X306_Panel (Autodesk Fusion 360 design; units mm, degrees)
part number: 2026-07-25-11-08-38-963
Autodesk Fusion 360 part; units mm, degrees
note: some values were not read from the file. Chosen so that the rebuilt part matches the saved one: which bodies a step acts on.
sketch "Sketch197" plane through (0, 0, 0) normal (0, 0, 1) x (1, 0, 0)
  line L0 (-43.7, -31.15) -> (43.7, -31.15)
  line L1 (43.7, -31.15) -> (43.7, 31.15)
  line L2 (43.7, 31.15) -> (-43.7, 31.15)
  line L3 (-43.7, 31.15) -> (-43.7, -31.15)
extrude "Extrude197" add sketch "Sketch197" along normal blind 5 makes body 1
ref_plane "WorkPlane11" through (0, 0, 5) normal (0, 0, 1) x (1, 0, 0)
sketch "Sketch198" plane through (0, 0, 5) normal (0, 0, 1) x (1, 0, 0)
  line L0 (-38.7, -26.15) -> (38.7, -26.15)
  line L1 (38.7, -26.15) -> (38.7, 26.15)
  line L2 (38.7, 26.15) -> (-38.7, 26.15)
  line L3 (-38.7, 26.15) -> (-38.7, -26.15)
extrude "Extrude198" cut sketch "Sketch198" against normal blind 2 bodies 1
sketch "Sketch199" plane through (0, 0, 0) normal (0, 0, 1) x (1, 0, 0)
  circle A0 centre (-35.05, 0.5) radius 1.55
extrude "Extrude199" cut sketch "Sketch199" along normal blind 6 bodies 1
sketch "Sketch200" plane through (0, 0, 0) normal (0, 0, 1) x (1, 0, 0)
  circle A0 centre (-35.05, -22.5) radius 1.55
extrude "Extrude200" cut sketch "Sketch200" along normal blind 6 bodies 1
sketch "Sketch201" plane through (0, 0, 0) normal (0, 0, 1) x (1, 0, 0)
  circle A0 centre (22.95, 0.5) radius 1.55
extrude "Extrude201" cut sketch "Sketch201" along normal blind 6 bodies 1
sketch "Sketch202" plane through (0, 0, 0) normal (0, 0, 1) x (1, 0, 0)
  circle A0 centre (22.95, -22.5) radius 1.55
extrude "Extrude202" cut sketch "Sketch202" along normal blind 6 bodies 1
ref_plane "WorkPlane12" through (0, 0, 5) normal (0, 0, 1) x (1, 0, 0)
sketch "Sketch203" plane through (0, 0, 5) normal (0, 0, 1) x (1, 0, 0)
  line L0 (-44.7, -16.03) -> (-38.7, -16.03)
  line L1 (-38.7, -16.03) -> (-38.7, -8.03)
  line L2 (-38.7, -8.03) -> (-44.7, -8.03)
  line L3 (-44.7, -8.03) -> (-44.7, -16.03)
extrude "Extrude203" cut sketch "Sketch203" against normal blind 2 bodies 1
ref_plane "WorkPlane13" through (0, 0, 1.4) normal (0, 0, 1) x (1, 0, 0)
sketch "Sketch204" plane through (0, 0, 0) normal (0, 0, 1) x (1, 0, 0)
  circle A0 centre (-35.05, 0.5) radius 2.95
sketch "Sketch205" plane through (0, 0, 1.4) normal (0, 0, 1) x (1, 0, 0)
  circle A0 centre (-35.05, 0.5) radius 1.55
loft "Loft1" cut profiles "Sketch204", "Sketch205" section 1 section 2 bodies 1
sketch "Sketch206" plane through (0, 0, 0) normal (0, 0, 1) x (1, 0, 0)
  circle A0 centre (-35.05, -22.5) radius 2.95
sketch "Sketch207" plane through (0, 0, 1.4) normal (0, 0, 1) x (1, 0, 0)
  circle A0 centre (-35.05, -22.5) radius 1.55
loft "Loft2" cut profiles "Sketch206", "Sketch207" section 1 section 2 bodies 1
sketch "Sketch208" plane through (0, 0, 0) normal (0, 0, 1) x (1, 0, 0)
  circle A0 centre (22.95, 0.5) radius 2.95
sketch "Sketch209" plane through (0, 0, 1.4) normal (0, 0, 1) x (1, 0, 0)
  circle A0 centre (22.95, 0.5) radius 1.55
loft "Loft3" cut profiles "Sketch208", "Sketch209" section 1 section 2 bodies 1
sketch "Sketch210" plane through (0, 0, 0) normal (0, 0, 1) x (1, 0, 0)
  circle A0 centre (22.95, -22.5) radius 2.95
sketch "Sketch211" plane through (0, 0, 1.4) normal (0, 0, 1) x (1, 0, 0)
  circle A0 centre (22.95, -22.5) radius 1.55
loft "Loft4" cut profiles "Sketch210", "Sketch211" section 1 section 2 bodies 1
ref_plane "WorkPlane14" through (0, 0, 5) normal (0, 0, 1) x (1, 0, 0)
sketch "Sketch212" plane through (0, 0, 5) normal (0, 0, 1) x (1, 0, 0)
  line L0 (27.25, -32.15) -> (37.25, -32.15)
  line L1 (37.25, -32.15) -> (37.25, -26.15)
  line L2 (37.25, -26.15) -> (27.25, -26.15)
  line L3 (27.25, -26.15) -> (27.25, -32.15)
extrude "Extrude204" cut sketch "Sketch212" against normal blind 2 bodies 1
ref_plane "WorkPlane15" through (0, 0, 3) normal (0, 0, 1) x (1, 0, 0)
sketch "Sketch213" plane through (0, 0, 3) normal (0, 0, 1) x (1, 0, 0)
  circle A0 centre (-36.405, 15.35) radius 1
extrude "Extrude205" cut sketch "Sketch213" against normal blind 2 bodies 1
sketch "Sketch214" plane through (0, 0, 3) normal (0, 0, 1) x (1, 0, 0)
  circle A0 centre (36.405, 15.35) radius 1
extrude "Extrude206" cut sketch "Sketch214" against normal blind 2 bodies 1
ref_plane "WorkPlane16" through (0, 0, 3) normal (0, 0, 1) x (1, 0, 0)
sketch "Sketch215" plane through (0, 0, 3) normal (0, 0, 1) x (1, 0, 0)
  circle A0 centre (-27.6, 7.35) radius 1.825
extrude "Extrude207" cut sketch "Sketch215" against normal blind 2 bodies 1
sketch "Sketch216" plane through (0, 0, 3) normal (0, 0, 1) x (1, 0, 0)
  circle A0 centre (27.6, 23.35) radius 1.825
extrude "Extrude208" cut sketch "Sketch216" against normal blind 2 bodies 1
ref_plane "WorkPlane17" through (0, 0, 5) normal (0, 0, 1) x (1, 0, 0)
sketch "Sketch217" plane through (0, 0, 5) normal (0, 0, 1) x (1, 0, 0)
  line L0 (-43.7, -31.15) -> (43.7, -31.15)
  line L1 (43.7, -31.15) -> (43.7, 31.15)
  line L2 (43.7, 31.15) -> (-43.7, 31.15)
  line L3 (-43.7, 31.15) -> (-43.7, -31.15)
extrude "Extrude209" add sketch "Sketch217" along normal blind 20 separate body makes body 2
sketch "Sketch218" plane through (0, 0, 5) normal (0, 0, 1) x (1, 0, 0)
  line L0 (-38.7, -26.15) -> (38.7, -26.15)
  line L1 (38.7, -26.15) -> (38.7, 26.15)
  line L2 (38.7, 26.15) -> (-38.7, 26.15)
  line L3 (-38.7, 26.15) -> (-38.7, -26.15)
extrude "Extrude210" cut sketch "Sketch218" along normal blind 20 bodies 2
sketch "Sketch219" plane through (0, 0, 5) normal (0, 0, 1) x (1, 0, 0)
  line L0 (-44.7, -16.03) -> (-37.7, -16.03)
  line L1 (-37.7, -16.03) -> (-37.7, -8.03)
  line L2 (-37.7, -8.03) -> (-44.7, -8.03)
  line L3 (-44.7, -8.03) -> (-44.7, -16.03)
extrude "Extrude211" cut sketch "Sketch219" along normal blind 20 bodies 2
sketch "Sketch220" plane through (0, 0, 5) normal (0, 0, 1) x (1, 0, 0)
  line L0 (27.25, -32.65) -> (37.25, -32.65)
  line L1 (37.25, -32.65) -> (37.25, -25.65)
  line L2 (37.25, -25.65) -> (27.25, -25.65)
  line L3 (27.25, -25.65) -> (27.25, -32.65)
extrude "Extrude212" cut sketch "Sketch220" along normal blind 20 bodies 2 makes body 3 at (-20.05, -31.15, 18.3333)
combine "Combine8" operation add target body 1 tool bodies 2
combine "Combine9" operation add target body 1 tool bodies 3
ref_plane "WorkPlane18" through (0, 0, 3) normal (0, 0, 1) x (1, 0, 0)
sketch "Sketch221" plane through (0, 0, 3) normal (0, 0, 1) x (1, 0, 0)
  line L0 (25.25, -32.15) -> (39.25, -32.15)
  line L1 (39.25, -32.15) -> (39.25, -26.15)
  line L2 (39.25, -26.15) -> (25.25, -26.15)
  line L3 (25.25, -26.15) -> (25.25, -32.15)
extrude "Extrude213" cut sketch "Sketch221" along normal blind 22 bodies 1
ref_plane "WorkPlane19" through (0, 0, 9) normal (0, 0, 1) x (1, 0, 0)
sketch "Sketch222" plane through (0, 0, 9) normal (0, 0, 1) x (1, 0, 0)
  line L0 (-43.7, -16.03) -> (-38.7, -16.03)
  line L1 (-38.7, -16.03) -> (-38.7, -8.03)
  line L2 (-38.7, -8.03) -> (-43.7, -8.03)
  line L3 (-43.7, -8.03) -> (-43.7, -16.03)
extrude "Extrude214" add sketch "Sketch222" along normal blind 16 separate body makes body 4
ref_plane "WorkPlane20" through (0, 0, 11) normal (0, 0, 1) x (1, 0, 0)
sketch "Sketch223" plane through (0, 0, 11) normal (0, 0, 1) x (1, 0, 0)
  line L0 (25.25, -31.15) -> (39.25, -31.15)
  line L1 (39.25, -31.15) -> (39.25, -26.15)
  line L2 (39.25, -26.15) -> (25.25, -26.15)
  line L3 (25.25, -26.15) -> (25.25, -31.15)
extrude "Extrude215" add sketch "Sketch223" along normal blind 14 separate body makes body 5
combine "Combine10" operation add target body 1 tool bodies 4 5
ref_plane "WorkPlane21" through (0, 0, 3) normal (0, 0, 1) x (1, 0, 0)
sketch "Sketch224" plane through (0, 0, 3) normal (0, 0, 1) x (1, 0, 0)
  line L0 (-38.7, -26.15) -> (-35.5, -26.15)
  line L1 (-35.5, -26.15) -> (-38.7, -22.95)
  line L2 (-38.7, -22.95) -> (-38.7, -26.15)
extrude "Extrude216" cut sketch "Sketch224" along normal blind 22 bodies 1
sketch "Sketch225" plane through (0, 0, 3) normal (0, 0, 1) x (1, 0, 0)
  line L0 (38.7, -26.15) -> (35.5, -26.15)
  line L1 (35.5, -26.15) -> (38.7, -22.95)
  line L2 (38.7, -22.95) -> (38.7, -26.15)
extrude "Extrude217" cut sketch "Sketch225" along normal blind 22 bodies 1
sketch "Sketch226" plane through (0, 0, 3) normal (0, 0, 1) x (1, 0, 0)
  line L0 (-38.7, 26.15) -> (-38, 26.15)
  line L1 (-38, 26.15) -> (-38.7, 25.45)
  line L2 (-38.7, 25.45) -> (-38.7, 26.15)
extrude "Extrude218" cut sketch "Sketch226" along normal blind 22 bodies 1
sketch "Sketch227" plane through (0, 0, 3) normal (0, 0, 1) x (1, 0, 0)
  line L0 (38.7, 26.15) -> (38, 26.15)
  line L1 (38, 26.15) -> (38.7, 25.45)
  line L2 (38.7, 25.45) -> (38.7, 26.15)
extrude "Extrude219" cut sketch "Sketch227" along normal blind 22 bodies 1
ref_plane "WorkPlane22" through (0, 0, 5) normal (0, 0, 1) x (1, 0, 0)
sketch "Sketch228" plane through (0, 0, 5) normal (0, 0, 1) x (1, 0, 0)
  line L0 (-44.7, -31.15) -> (44.7, -31.15)
  line L1 (44.7, -31.15) -> (44.7, -26.15)
  line L2 (44.7, -26.15) -> (-44.7, -26.15)
  line L3 (-44.7, -26.15) -> (-44.7, -31.15)
extrude "Extrude220" cut sketch "Sketch228" along normal blind 20 bodies 1
ref_plane "WorkPlane23" through (0, 0, 5) normal (0, 0, 1) x (1, 0, 0)
sketch "Sketch229" plane through (0, 0, 5) normal (0, 0, 1) x (1, 0, 0)
  line L0 (-43.7, -31.15) -> (-38.7, -31.15)
  line L1 (-38.7, -31.15) -> (-38.7, -26.15)
  line L2 (-38.7, -26.15) -> (-43.7, -26.15)
  line L3 (-43.7, -26.15) -> (-43.7, -31.15)
extrude "Extrude221" add sketch "Sketch229" along normal blind 20 separate body makes body 6
sketch "Sketch230" plane through (0, 0, 5) normal (0, 0, 1) x (1, 0, 0)
  line L0 (38.7, -31.15) -> (43.7, -31.15)
  line L1 (43.7, -31.15) -> (43.7, -26.15)
  line L2 (43.7, -26.15) -> (38.7, -26.15)
  line L3 (38.7, -26.15) -> (38.7, -31.15)
extrude "Extrude222" add sketch "Sketch230" along normal blind 20 separate body makes body 7
combine "Combine11" operation add target body 1 tool bodies 6 7
ref_plane "WorkPlane24" through (0, 0, 3) normal (0, 0, 1) x (1, 0, 0)
sketch "Sketch231" plane through (0, 0, 3) normal (0, 0, 1) x (1, 0, 0)
  line L0 (-43.7, -16.03) -> (-38.7, -16.03)
  line L1 (-38.7, -16.03) -> (-38.7, -8.03)
  line L2 (-38.7, -8.03) -> (-43.7, -8.03)
  line L3 (-43.7, -8.03) -> (-43.7, -16.03)
extrude "Extrude223" add sketch "Sketch231" along normal blind 6 separate body makes body 8
combine "Combine12" operation add target body 1 tool bodies 8
ref_plane "WorkPlane25" through (-43.7, 0, 0) normal (1, 0, 0) x (0, 1, 0)
sketch "Sketch232" plane through (-43.7, 0, 0) normal (1, 0, 0) x (0, 0, -1)
  circle A0 centre (-6, -16.5) radius 3.2
extrude "Extrude224" cut sketch "Sketch232" along normal blind 5.2 bodies 1
sketch "Sketch233" plane through (0, 0, 0) normal (0, 0, 1) x (1, 0, 0)
  line L0 (-49.7, -37.15) -> (-43.7, -37.15)
  line L1 (-43.7, -37.15) -> (-43.7, 37.15)
  line L2 (-43.7, 37.15) -> (-49.7, 37.15)
  line L3 (-49.7, 37.15) -> (-49.7, -37.15)
extrude "Extrude225" add sketch "Sketch233" along normal blind 25 separate body makes body 9
sketch "Sketch234" plane through (0, 0, 0) normal (0, 0, 1) x (1, 0, 0)
  line L0 (43.7, -37.15) -> (49.7, -37.15)
  line L1 (49.7, -37.15) -> (49.7, 37.15)
  line L2 (49.7, 37.15) -> (43.7, 37.15)
  line L3 (43.7, 37.15) -> (43.7, -37.15)
extrude "Extrude226" add sketch "Sketch234" along normal blind 25 separate body makes body 10
sketch "Sketch235" plane through (0, 0, 0) normal (0, 0, 1) x (1, 0, 0)
  line L0 (-43.7, 31.15) -> (43.7, 31.15)
  line L1 (43.7, 31.15) -> (43.7, 37.15)
  line L2 (43.7, 37.15) -> (-43.7, 37.15)
  line L3 (-43.7, 37.15) -> (-43.7, 31.15)
extrude "Extrude227" add sketch "Sketch235" along normal blind 25 separate body makes body 11
sketch "Sketch236" plane through (0, 0, 0) normal (0, 0, 1) x (1, 0, 0)
  line L0 (-43.7, -37.15) -> (43.7, -37.15)
  line L1 (43.7, -37.15) -> (43.7, -31.15)
  line L2 (43.7, -31.15) -> (-43.7, -31.15)
  line L3 (-43.7, -31.15) -> (-43.7, -37.15)
extrude "Extrude228" add sketch "Sketch236" along normal blind 5 separate body makes body 12
combine "Combine13" operation add target body 1 tool bodies 9 10 11 12
ref_plane "WorkPlane27" through (-49.7, 0, 0) normal (1, 0, 0) x (0, 1, 0)
sketch "Sketch238" plane through (-49.7, 0, 0) normal (1, 0, 0) x (0, 0, -1)
  circle A0 centre (-6, -16.5) radius 3.2
extrude "Extrude229" cut sketch "Sketch238" along normal blind 11.3 bodies 1
ref_plane "WorkPlane28" through (0, -37.15, 0) normal (0, 1, 0) x (0, 0, 1)
sketch "Sketch239" plane through (0, -37.15, 0) normal (0, 1, 0) x (1, 0, 0)
  line L0 (25.25, -5) -> (39.25, -5)
  line L1 (39.25, -5) -> (39.25, -3)
  line L2 (39.25, -3) -> (25.25, -3)
  line L3 (25.25, -3) -> (25.25, -5)
extrude "Extrude230" cut sketch "Sketch239" along normal blind 11.2 bodies 1
sketch "Sketch240" plane through (0, 0, 0) normal (0, 0, 1) x (1, 0, 0)
  line L0 (38.7, -37.15) -> (49.7, -37.15)
  line L1 (49.7, -37.15) -> (49.7, -26.15)
  line L2 (49.7, -26.15) -> (38.7, -26.15)
  line L3 (38.7, -26.15) -> (38.7, -37.15)
  line L4 (-49.7, -37.15) -> (-38.7, -37.15)
  line L5 (-38.7, -37.15) -> (-38.7, -26.15)
  line L6 (-38.7, -26.15) -> (-49.7, -26.15)
  line L7 (-49.7, -26.15) -> (-49.7, -37.15)
extrude "Extrude231" add sketch "Sketch240" along normal blind 25 separate body makes body 13 at (46.0333, -26.15, 8.3333) makes body 14 at (-42.3667, -26.15, 8.3333)
combine "Combine14" operation add target body 1 tool bodies 13 14
ref_plane "WorkPlane29" through (0, -37.15, 0) normal (0, 1, 0) x (0, 0, 1)
sketch "Sketch241" plane through (0, -37.15, 0) normal (0, 1, 0) x (1, 0, 0)
  line L0 (25.25, -5) -> (39.25, -5)
  line L1 (39.25, -5) -> (39.25, -3)
  line L2 (39.25, -3) -> (25.25, -3)
  line L3 (25.25, -3) -> (25.25, -5)
extrude "Extrude232" cut sketch "Sketch241" along normal blind 11.2 bodies 1
sketch "Sketch242" plane through (0, 0, 0) normal (0, 0, 1) x (1, 0, 0)
  circle A0 centre (-44.2, 31.65) radius 1.7
  circle A1 centre (44.2, 31.65) radius 1.7
  circle A2 centre (-44.2, -31.65) radius 1.7
  circle A3 centre (44.2, -31.65) radius 1.7
extrude "Extrude233" cut sketch "Sketch242" along normal blind 25 bodies 1
sketch "Sketch243" plane through (0, 0, 0) normal (0, 0, 1) x (1, 0, 0)
  line L0 (-40.9091, 31.65) -> (-42.5546, 34.5)
  line L1 (-42.5546, 34.5) -> (-45.8454, 34.5)
  line L2 (-45.8454, 34.5) -> (-47.4909, 31.65)
  line L3 (-47.4909, 31.65) -> (-45.8454, 28.8)
  line L4 (-45.8454, 28.8) -> (-42.5546, 28.8)
  line L5 (-42.5546, 28.8) -> (-40.9091, 31.65)
  line L6 (47.4909, 31.65) -> (45.8454, 34.5)
  line L7 (45.8454, 34.5) -> (42.5546, 34.5)
  line L8 (42.5546, 34.5) -> (40.9091, 31.65)
  line L9 (40.9091, 31.65) -> (42.5546, 28.8)
  line L10 (42.5546, 28.8) -> (45.8454, 28.8)
  line L11 (45.8454, 28.8) -> (47.4909, 31.65)
  line L12 (-40.9091, -31.65) -> (-42.5546, -28.8)
  line L13 (-42.5546, -28.8) -> (-45.8454, -28.8)
  line L14 (-45.8454, -28.8) -> (-47.4909, -31.65)
  line L15 (-47.4909, -31.65) -> (-45.8454, -34.5)
  line L16 (-45.8454, -34.5) -> (-42.5546, -34.5)
  line L17 (-42.5546, -34.5) -> (-40.9091, -31.65)
  line L18 (47.4909, -31.65) -> (45.8454, -28.8)
  line L19 (45.8454, -28.8) -> (42.5546, -28.8)
  line L20 (42.5546, -28.8) -> (40.9091, -31.65)
  line L21 (40.9091, -31.65) -> (42.5546, -34.5)
  line L22 (42.5546, -34.5) -> (45.8454, -34.5)
  line L23 (45.8454, -34.5) -> (47.4909, -31.65)
extrude "Extrude234" cut sketch "Sketch243" along normal blind 2.6 bodies 1
ref_plane "WorkPlane30" through (0, 0, 15) normal (0, 0, 1) x (1, 0, 0)
sketch "Sketch244" plane through (0, 0, 15) normal (0, 0, 1) x (1, 0, 0)
  line L0 (-60, -50) -> (60, -50)
  line L1 (60, -50) -> (60, 50)
  line L2 (60, 50) -> (-60, 50)
  line L3 (-60, 50) -> (-60, -50)
extrude "Extrude235" cut sketch "Sketch244" along normal blind 15 bodies 1
sketch "Sketch245" plane through (0, 0, 0) normal (0, 0, 1) x (1, 0, 0)
  line L0 (-49.7, -37.15, 15) -> (-38.7, -37.15, 15)
  line L1 (-38.7, -37.15, 15) -> (-38.7, 37.15, 15)
  line L2 (-38.7, 37.15, 15) -> (-49.7, 37.15, 15)
  line L3 (-49.7, 37.15, 15) -> (-49.7, -37.15, 15)
sketch "Sketch245 (curves 15 mm off its plane)" plane through (0, 0, 15) normal (0, 0, 1) x (1, 0, 0)
  line L0 (-49.7, -37.15) -> (-38.7, -37.15)
  line L1 (-38.7, -37.15) -> (-38.7, 37.15)
  line L2 (-38.7, 37.15) -> (-49.7, 37.15)
  line L3 (-49.7, 37.15) -> (-49.7, -37.15)
extrude "Extrude236" add sketch "Sketch245 (curves 15 mm off its plane)" along normal blind 32 separate body makes body 15
sketch "Sketch246" plane through (0, 0, 0) normal (0, 0, 1) x (1, 0, 0)
  line L0 (38.7, -37.15, 15) -> (49.7, -37.15, 15)
  line L1 (49.7, -37.15, 15) -> (49.7, 37.15, 15)
  line L2 (49.7, 37.15, 15) -> (38.7, 37.15, 15)
  line L3 (38.7, 37.15, 15) -> (38.7, -37.15, 15)
sketch "Sketch246 (curves 15 mm off its plane)" plane through (0, 0, 15) normal (0, 0, 1) x (1, 0, 0)
  line L0 (38.7, -37.15) -> (49.7, -37.15)
  line L1 (49.7, -37.15) -> (49.7, 37.15)
  line L2 (49.7, 37.15) -> (38.7, 37.15)
  line L3 (38.7, 37.15) -> (38.7, -37.15)
extrude "Extrude237" add sketch "Sketch246 (curves 15 mm off its plane)" along normal blind 32 separate body makes body 16
sketch "Sketch247" plane through (0, 0, 0) normal (0, 0, 1) x (1, 0, 0)
  line L0 (-38.7, 26.15, 15) -> (38.7, 26.15, 15)
  line L1 (38.7, 26.15, 15) -> (38.7, 37.15, 15)
  line L2 (38.7, 37.15, 15) -> (-38.7, 37.15, 15)
  line L3 (-38.7, 37.15, 15) -> (-38.7, 26.15, 15)
sketch "Sketch247 (curves 15 mm off its plane)" plane through (0, 0, 15) normal (0, 0, 1) x (1, 0, 0)
  line L0 (-38.7, 26.15) -> (38.7, 26.15)
  line L1 (38.7, 26.15) -> (38.7, 37.15)
  line L2 (38.7, 37.15) -> (-38.7, 37.15)
  line L3 (-38.7, 37.15) -> (-38.7, 26.15)
extrude "Extrude238" add sketch "Sketch247 (curves 15 mm off its plane)" along normal blind 32 separate body makes body 17
sketch "Sketch248" plane through (0, 0, 0) normal (0, 0, 1) x (1, 0, 0)
  line L0 (-49.7, -37.15, 47) -> (49.7, -37.15, 47)
  line L1 (49.7, -37.15, 47) -> (49.7, 37.15, 47)
  line L2 (49.7, 37.15, 47) -> (-49.7, 37.15, 47)
  line L3 (-49.7, 37.15, 47) -> (-49.7, -37.15, 47)
sketch "Sketch248 (curves 47 mm off its plane)" plane through (0, 0, 47) normal (0, 0, 1) x (1, 0, 0)
  line L0 (-49.7, -37.15) -> (49.7, -37.15)
  line L1 (49.7, -37.15) -> (49.7, 37.15)
  line L2 (49.7, 37.15) -> (-49.7, 37.15)
  line L3 (-49.7, 37.15) -> (-49.7, -37.15)
extrude "Extrude239" add sketch "Sketch248 (curves 47 mm off its plane)" along normal blind 3 separate body makes body 18
combine "Combine15" operation add target body 15 tool bodies 16 17 18
sketch "Sketch249" plane through (0, 0, 0) normal (0, 0, 1) x (1, 0, 0)
  line L0 (-12, -7, 47) -> (12, -7, 47)
  line L1 (12, -7, 47) -> (12, 7, 47)
  line L2 (12, 7, 47) -> (-12, 7, 47)
  line L3 (-12, 7, 47) -> (-12, -7, 47)
sketch "Sketch249 (curves 47 mm off its plane)" plane through (0, 0, 47) normal (0, 0, 1) x (1, 0, 0)
  line L0 (-12, -7) -> (12, -7)
  line L1 (12, -7) -> (12, 7)
  line L2 (12, 7) -> (-12, 7)
  line L3 (-12, 7) -> (-12, -7)
extrude "Extrude240" cut sketch "Sketch249 (curves 47 mm off its plane)" along normal blind 3 bodies 15
sketch "Sketch250" plane through (0, 0, 0) normal (0, 0, 1) x (1, 0, 0)
  circle A0 through (-42.5, 31.65, 15) (-45.05, 33.1222, 15) (-45.05, 30.1778, 15)
  circle A1 through (45.9, 31.65, 15) (43.35, 33.1222, 15) (43.35, 30.1778, 15)
  circle A2 through (-42.5, -31.65, 15) (-45.05, -30.1778, 15) (-45.05, -33.1222, 15)
  circle A3 through (45.9, -31.65, 15) (43.35, -30.1778, 15) (43.35, -33.1222, 15)
sketch "Sketch250 (curves 15 mm off its plane)" plane through (0, 0, 15) normal (0, 0, 1) x (1, 0, 0)
  circle A0 centre (-44.2, 31.65) radius 1.7
  circle A1 centre (44.2, 31.65) radius 1.7
  circle A2 centre (-44.2, -31.65) radius 1.7
  circle A3 centre (44.2, -31.65) radius 1.7
extrude "Extrude241" cut sketch "Sketch250 (curves 15 mm off its plane)" along normal blind 35 bodies 15
sketch "Sketch251" plane through (0, 0, 0) normal (0, 0, 1) x (1, 0, 0)
  circle A0 through (-41.1, 31.65, 50) (-45.75, 34.3347, 50) (-45.75, 28.9653, 50)
sketch "Sketch252" plane through (0, 0, 0) normal (0, 0, 1) x (1, 0, 0)
  circle A0 through (-42.5, 31.65, 48.2) (-45.05, 33.1222, 48.2) (-45.05, 30.1778, 48.2)
sketch "Sketch251 (curves 50 mm off its plane)" plane through (0, 0, 50) normal (0, 0, 1) x (1, 0, 0)
  circle A0 centre (-44.2, 31.65) radius 3.1
sketch "Sketch252 (curves 48.2 mm off its plane)" plane through (0, 0, 48.2) normal (0, 0, 1) x (1, 0, 0)
  circle A0 centre (-44.2, 31.65) radius 1.7
loft "Loft5" cut profiles "Sketch251 (curves 50 mm off its plane)", "Sketch252 (curves 48.2 mm off its plane)" section 1 section 2 bodies 15
sketch "Sketch253" plane through (0, 0, 0) normal (0, 0, 1) x (1, 0, 0)
  circle A0 through (47.3, 31.65, 50) (42.65, 34.3347, 50) (42.65, 28.9653, 50)
sketch "Sketch254" plane through (0, 0, 0) normal (0, 0, 1) x (1, 0, 0)
  circle A0 through (45.9, 31.65, 48.2) (43.35, 33.1222, 48.2) (43.35, 30.1778, 48.2)
sketch "Sketch253 (curves 50 mm off its plane)" plane through (0, 0, 50) normal (0, 0, 1) x (1, 0, 0)
  circle A0 centre (44.2, 31.65) radius 3.1
sketch "Sketch254 (curves 48.2 mm off its plane)" plane through (0, 0, 48.2) normal (0, 0, 1) x (1, 0, 0)
  circle A0 centre (44.2, 31.65) radius 1.7
loft "Loft6" cut profiles "Sketch253 (curves 50 mm off its plane)", "Sketch254 (curves 48.2 mm off its plane)" section 1 section 2 bodies 15
sketch "Sketch255" plane through (0, 0, 0) normal (0, 0, 1) x (1, 0, 0)
  circle A0 through (-41.1, -31.65, 50) (-45.75, -28.9653, 50) (-45.75, -34.3347, 50)
sketch "Sketch256" plane through (0, 0, 0) normal (0, 0, 1) x (1, 0, 0)
  circle A0 through (-42.5, -31.65, 48.2) (-45.05, -30.1778, 48.2) (-45.05, -33.1222, 48.2)
sketch "Sketch255 (curves 50 mm off its plane)" plane through (0, 0, 50) normal (0, 0, 1) x (1, 0, 0)
  circle A0 centre (-44.2, -31.65) radius 3.1
sketch "Sketch256 (curves 48.2 mm off its plane)" plane through (0, 0, 48.2) normal (0, 0, 1) x (1, 0, 0)
  circle A0 centre (-44.2, -31.65) radius 1.7
loft "Loft7" cut profiles "Sketch255 (curves 50 mm off its plane)", "Sketch256 (curves 48.2 mm off its plane)" section 1 section 2 bodies 15
sketch "Sketch257" plane through (0, 0, 0) normal (0, 0, 1) x (1, 0, 0)
  circle A0 through (47.3, -31.65, 50) (42.65, -28.9653, 50) (42.65, -34.3347, 50)
sketch "Sketch258" plane through (0, 0, 0) normal (0, 0, 1) x (1, 0, 0)
  circle A0 through (45.9, -31.65, 48.2) (43.35, -30.1778, 48.2) (43.35, -33.1222, 48.2)
sketch "Sketch257 (curves 50 mm off its plane)" plane through (0, 0, 50) normal (0, 0, 1) x (1, 0, 0)
  circle A0 centre (44.2, -31.65) radius 3.1
sketch "Sketch258 (curves 48.2 mm off its plane)" plane through (0, 0, 48.2) normal (0, 0, 1) x (1, 0, 0)
  circle A0 centre (44.2, -31.65) radius 1.7
loft "Loft8" cut profiles "Sketch257 (curves 50 mm off its plane)", "Sketch258 (curves 48.2 mm off its plane)" section 1 section 2 bodies 15
sketch "Sketch259" plane through (0, 0, 0) normal (0, 0, 1) x (1, 0, 0)
  circle A0 through (-8.75, -10.75, 47) (-11.75, -9.0179, 47) (-11.75, -12.4821, 47)
  circle A1 through (12.75, -10.75, 47) (9.75, -9.0179, 47) (9.75, -12.4821, 47)
  circle A2 through (-8.75, 10.75, 47) (-11.75, 12.4821, 47) (-11.75, 9.0179, 47)
  circle A3 through (12.75, 10.75, 47) (9.75, 12.4821, 47) (9.75, 9.0179, 47)
sketch "Sketch259 (curves 47 mm off its plane)" plane through (0, 0, 47) normal (0, 0, 1) x (1, 0, 0)
  circle A0 centre (-10.75, -10.75) radius 2
  circle A1 centre (10.75, -10.75) radius 2
  circle A2 centre (-10.75, 10.75) radius 2
  circle A3 centre (10.75, 10.75) radius 2
extrude "Extrude242" add sketch "Sketch259 (curves 47 mm off its plane)" against normal blind 4 separate body makes body 19 at (-8.7599, 10.5509, 45.6667) makes body 20 at (12.7401, -10.9491, 45.6667) makes body 21 at (-8.7599, -10.9491, 45.6667) makes body 22 at (12.7401, 10.5509, 45.6667)
combine "Combine16" operation add target body 15 tool bodies 19 20 21 22
sketch "Sketch260" plane through (0, 0, 0) normal (0, 0, 1) x (1, 0, 0)
  circle A0 through (-9.95, -10.75, 47) (-11.15, -10.0572, 47) (-11.15, -11.4428, 47)
  circle A1 through (11.55, -10.75, 47) (10.35, -10.0572, 47) (10.35, -11.4428, 47)
  circle A2 through (-9.95, 10.75, 47) (-11.15, 11.4428, 47) (-11.15, 10.0572, 47)
  circle A3 through (11.55, 10.75, 47) (10.35, 11.4428, 47) (10.35, 10.0572, 47)
sketch "Sketch260 (curves 47 mm off its plane)" plane through (0, 0, 47) normal (0, 0, 1) x (1, 0, 0)
  circle A0 centre (-10.75, -10.75) radius 0.8
  circle A1 centre (10.75, -10.75) radius 0.8
  circle A2 centre (-10.75, 10.75) radius 0.8
  circle A3 centre (10.75, 10.75) radius 0.8
extrude "Extrude243" cut sketch "Sketch260 (curves 47 mm off its plane)" against normal blind 4 bodies 15
named bodies: "RingWest", "RingEast", "RingNorth", "RingSouth", "TopPart", "TopRingEast", "TopRingNorth", "TopRoof"
